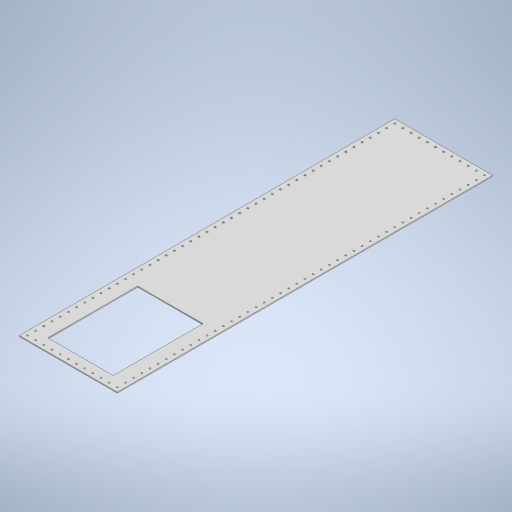
# Autodesk Inventor part: BOTTOM DS new
Saved by Autodesk Inventor 2023.4 (Build 274418000, 418)
## iProperties
Created: 2023-12-21
Part Number: BOTTOM DS new
Material: Generic
Document SubType Name: Sheet Metal
Designer: elija
Density: 1 g/cm^3
Sheet Metal Rule: Default
Appearance: Default
Author: elija
Autodesk Inventor part; units mm, degrees
ref_plane "YZ Plane" through (0, 0, 0) normal (1, 0, 0) x (0, 1, 0)
ref_plane "XZ Plane" through (0, 0, 0) normal (0, 1, 0) x (-1, 0, 0)
ref_plane "XY Plane" through (0, 0, 0) normal (0, 0, 1) x (1, 0, 0)
sketch "Sketch1" plane through (0, 0, 0) normal (0, 1, 0) x (-1, 0, 0)
  line L0 (0, 0) -> (304.8, 0)
  line L1 (304.8, 0) -> (304.8, -1168.4)
  line L2 (304.8, -1168.4) -> (0, -1168.4)
  line L3 (0, -1168.4) -> (0, 0)
  circle A0 centre (292.1, -12.7) radius 2.5019
  circle A1 centre (12.7, -12.7) radius 2.5019
  circle A2 centre (38.1, -12.7) radius 2.5019
  circle A3 centre (63.5, -12.7) radius 2.5019
  circle A4 centre (88.9, -12.7) radius 2.5019
  circle A5 centre (114.3, -12.7) radius 2.5019
  circle A6 centre (139.7, -12.7) radius 2.5019
  circle A7 centre (165.1, -12.7) radius 2.5019
  circle A8 centre (190.5, -12.7) radius 2.5019
  circle A9 centre (215.9, -12.7) radius 2.5019
  circle A10 centre (241.3, -12.7) radius 2.5019
  circle A11 centre (266.7, -12.7) radius 2.5019
  circle A12 centre (292.1, -12.7) radius 2.5019
  circle A13 centre (12.7, -38.1) radius 2.5019
  circle A14 centre (12.7, -63.5) radius 2.5019
  circle A15 centre (12.7, -88.9) radius 2.5019
  circle A16 centre (12.7, -114.3) radius 2.5019
  circle A17 centre (12.7, -139.7) radius 2.5019
  circle A18 centre (12.7, -165.1) radius 2.5019
  circle A19 centre (12.7, -190.5) radius 2.5019
  circle A20 centre (12.7, -215.9) radius 2.5019
  circle A21 centre (12.7, -241.3) radius 2.5019
  circle A22 centre (12.7, -266.7) radius 2.5019
  circle A23 centre (12.7, -292.1) radius 2.5019
  circle A24 centre (12.7, -317.5) radius 2.5019
  circle A25 centre (12.7, -342.9) radius 2.5019
  circle A26 centre (12.7, -368.3) radius 2.5019
  circle A27 centre (12.7, -393.7) radius 2.5019
  circle A28 centre (12.7, -419.1) radius 2.5019
  circle A29 centre (12.7, -444.5) radius 2.5019
  circle A30 centre (12.7, -469.9) radius 2.5019
  circle A31 centre (12.7, -495.3) radius 2.5019
  circle A32 centre (12.7, -520.7) radius 2.5019
  circle A33 centre (12.7, -546.1) radius 2.5019
  circle A34 centre (12.7, -571.5) radius 2.5019
  circle A35 centre (12.7, -596.9) radius 2.5019
  circle A36 centre (12.7, -622.3) radius 2.5019
  circle A37 centre (12.7, -647.7) radius 2.5019
  circle A38 centre (12.7, -673.1) radius 2.5019
  circle A39 centre (12.7, -698.5) radius 2.5019
  circle A40 centre (12.7, -723.9) radius 2.5019
  circle A41 centre (12.7, -749.3) radius 2.5019
  circle A42 centre (12.7, -774.7) radius 2.5019
  circle A43 centre (12.7, -800.1) radius 2.5019
  circle A44 centre (12.7, -825.5) radius 2.5019
  circle A45 centre (12.7, -850.9) radius 2.5019
  circle A46 centre (12.7, -876.3) radius 2.5019
  circle A47 centre (12.7, -901.7) radius 2.5019
  circle A48 centre (12.7, -927.1) radius 2.5019
  circle A49 centre (12.7, -952.5) radius 2.5019
  circle A50 centre (12.7, -977.9) radius 2.5019
  circle A51 centre (12.7, -1003.3) radius 2.5019
  circle A52 centre (12.7, -1028.7) radius 2.5019
  circle A53 centre (12.7, -1054.1) radius 2.5019
  circle A54 centre (12.7, -1079.5) radius 2.5019
  circle A55 centre (12.7, -1104.9) radius 2.5019
  circle A56 centre (12.7, -1130.3) radius 2.5019
  circle A57 centre (12.7, -1155.7) radius 2.5019
  circle A58 centre (38.1, -1155.7) radius 2.5019
  circle A59 centre (63.5, -1155.7) radius 2.5019
  circle A60 centre (88.9, -1155.7) radius 2.5019
  circle A61 centre (114.3, -1155.7) radius 2.5019
  circle A62 centre (139.7, -1155.7) radius 2.5019
  circle A63 centre (165.1, -1155.7) radius 2.5019
  circle A64 centre (190.5, -1155.7) radius 2.5019
  circle A65 centre (215.9, -1155.7) radius 2.5019
  circle A66 centre (241.3, -1155.7) radius 2.5019
  circle A67 centre (266.7, -1155.7) radius 2.5019
  circle A68 centre (292.1, -1155.7) radius 2.5019
  circle A69 centre (292.1, -1130.3) radius 2.5019
  circle A70 centre (292.1, -1104.9) radius 2.5019
  circle A71 centre (292.1, -1079.5) radius 2.5019
  circle A72 centre (292.1, -1054.1) radius 2.5019
  circle A73 centre (292.1, -1028.7) radius 2.5019
  circle A74 centre (292.1, -1003.3) radius 2.5019
  circle A75 centre (292.1, -977.9) radius 2.5019
  circle A76 centre (292.1, -952.5) radius 2.5019
  circle A77 centre (292.1, -927.1) radius 2.5019
  circle A78 centre (292.1, -901.7) radius 2.5019
  circle A79 centre (292.1, -876.3) radius 2.5019
  circle A80 centre (292.1, -850.9) radius 2.5019
  circle A81 centre (292.1, -825.5) radius 2.5019
  circle A82 centre (292.1, -800.1) radius 2.5019
  circle A83 centre (292.1, -774.7) radius 2.5019
  circle A84 centre (292.1, -749.3) radius 2.5019
  circle A85 centre (292.1, -723.9) radius 2.5019
  circle A86 centre (292.1, -698.5) radius 2.5019
  circle A87 centre (292.1, -673.1) radius 2.5019
  circle A88 centre (292.1, -647.7) radius 2.5019
  circle A89 centre (292.1, -622.3) radius 2.5019
  circle A90 centre (292.1, -596.9) radius 2.5019
  circle A91 centre (292.1, -571.5) radius 2.5019
  circle A92 centre (292.1, -546.1) radius 2.5019
  circle A93 centre (292.1, -520.7) radius 2.5019
  circle A94 centre (292.1, -495.3) radius 2.5019
  circle A95 centre (292.1, -469.9) radius 2.5019
  circle A96 centre (292.1, -444.5) radius 2.5019
  circle A97 centre (292.1, -419.1) radius 2.5019
  circle A98 centre (292.1, -393.7) radius 2.5019
  circle A99 centre (292.1, -368.3) radius 2.5019
  circle A100 centre (292.1, -342.9) radius 2.5019
  circle A101 centre (292.1, -317.5) radius 2.5019
  circle A102 centre (292.1, -292.1) radius 2.5019
  circle A103 centre (292.1, -266.7) radius 2.5019
  circle A104 centre (292.1, -241.3) radius 2.5019
  circle A105 centre (292.1, -215.9) radius 2.5019
  circle A106 centre (292.1, -190.5) radius 2.5019
  circle A107 centre (292.1, -165.1) radius 2.5019
  circle A108 centre (292.1, -139.7) radius 2.5019
  circle A109 centre (292.1, -114.3) radius 2.5019
  circle A110 centre (292.1, -88.9) radius 2.5019
  circle A111 centre (292.1, -63.5) radius 2.5019
  circle A112 centre (292.1, -38.1) radius 2.5019
  dimension "d0" = 1168.4
  dimension "d1" = 304.8
  dimension "d3" = 5.0038
  dimension "d4" = 12.7
  dimension "d5" = 12.7
  dimension "d6" = 5.0038
  dimension "d7" = 12.7
  dimension "d8" = 12.7
  dimension "d11" = 25.4
  dimension "d18" = 25.4
  dimension "d25" = 25.4
  dimension "d32" = 25.4
  constraints: 113 centre point, 8 end point, 3 horizontal, 2 parallel, 2 vertical, 1 perpendicular, 222 other
  measures "d0" distance of L0.end L1.end
  measures "d1" distance of L1.end L2.end
  measures "d3" diameter of A0
  measures "d4" distance from line of L0 A0.centre
  measures "d5" distance from line of L1 A0.centre
  measures "d6" diameter of A1
  measures "d7" distance from line of L0 A1.centre
  measures "d8" distance from line of L3 A1.centre
  measures "d11" distance of A1.centre A2.centre
  measures "d18" distance of A1.centre A13.centre
  measures "d25" distance of A57.centre A58.centre
  measures "d32" distance of A68.centre A69.centre
extrude "Plate2" add sketch "Sketch1" along normal blind 3.175
sketch "Sketch4" plane through (0, 3.175, 0) normal (0, 1, 0) x (1, 0, 0)
  line L0 (-254, 38.1) -> (-50.8, 38.1)
  line L1 (-50.8, 38.1) -> (-50.8, 317.5)
  line L2 (-50.8, 317.5) -> (-254, 317.5)
  line L3 (-254, 317.5) -> (-254, 38.1)
  line L4 (-304.8, 0) -> (-304.8, 1168.4) projected
  line L5 (0, 1168.4) -> (0, 0) projected
  line L6 (0, 0) -> (-304.8, 0) projected
  dimension "d83" = 203.2
  dimension "d84" = 279.4
  dimension "d85" = 50.8
  dimension "d86" = 50.8
  dimension "d87" = 38.1
  constraints: 8 end point, 2 parallel, 1 horizontal, 1 perpendicular
  measures "d83" distance of L2.end L1.end
  measures "d84" distance of L1.end L0.end
  measures "d85" distance between parallel lines of L4 L3
  measures "d86" distance between parallel lines of L5 L1
  measures "d87" distance between parallel lines of L6 L0
extrude "Extrusion6" cut sketch "Sketch4" against normal blind 25.4
equation "\"d37\" = Thickness"
equation "\"BendRadius\" = Thickness"
equation "\"BendReliefWidth\" = Thickness"
equation "\"BendReliefDepth\" = 0.5 * Thickness"
equation "\"CornerReliefSize\" = 4 * Thickness"
equation "\"MinimumRemnant\" = 2 * Thickness"
equation "\"TransitionRadius\" = BendRadius"
equation "\"JacobiRadiusSize\" = BendRadius"
equation "\"GapSize\" = Thickness"
equation "\"Thickness\" = 3.175"
body "Solid2"
